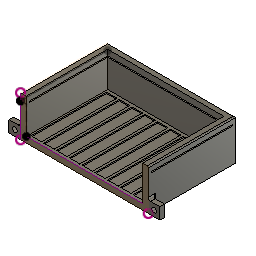
LIght box v2 (Autodesk Fusion 360 design; units mm, degrees)
Autodesk Fusion 360 part; units mm, degrees
sketch "Box base" plane through (0, 0, 0) normal (0, 1, 0) x (1, 0, 0)
  line L0 (55, -40) -> (-55, -40)
  line L1 (-55, -40) -> (-55, 40)
  line L2 (-55, 40) -> (55, 40)
  line L3 (55, 40) -> (55, -40)
  line L4 (55, -40) -> (-55, 40) construction
  line L5 (-55, -40) -> (55, 40) construction
  dimension "d3" = 110
  dimension "d4" = 80
extrude "Extrude2" add sketch "Box base" along normal blind 35
sketch "Center box" plane through (0, 35, 0) normal (0, 1, 0) x (-1, 0, 0)
  line L0 (-55, -40) -> (55, -40)
  line L1 (55, -40) -> (55, 40)
  line L2 (55, 40) -> (-55, 40)
  line L3 (-55, 40) -> (-55, -40)
  line L4 (-50, 35) -> (50, 35)
  line L5 (50, 35) -> (50, -35)
  line L6 (50, -35) -> (-50, -35)
  line L7 (-50, -35) -> (-50, 35)
  line L8 (-50, 35) -> (50, -35) construction
  line L9 (50, 35) -> (-50, -35) construction
  dimension "d9" = 100
  dimension "d10" = 70
extrude "Extrude3" cut sketch "Center box" against normal blind 30 contours L4 L5 L6 L7
sketch "open one end" plane through (0, 0, 40) normal (0, 0, 1) x (1, 0, 0)
  line L0 (-55, 0) -> (55, 0)
  line L1 (55, 0) -> (55, 35)
  line L2 (55, 35) -> (-55, 35)
  line L3 (-55, 35) -> (-55, 0)
  line L4 (-55, 35) -> (55, 35)
  line L5 (55, 35) -> (55, 0)
  line L6 (55, 0) -> (-55, 0)
  line L7 (-55, 0) -> (-55, 35)
extrude "Extrude4" cut sketch "open one end" against normal blind 5
sketch "line marker for slit" plane through (0, 0, 35) normal (0, 0, 1) x (1, 0, 0)
  line L0 (-50, 5) -> (-50, 35)
  line L1 (-50, 35) -> (-55, 35)
  line L2 (-55, 35) -> (-55, 0)
  line L3 (-55, 0) -> (55, 0)
  line L4 (55, 0) -> (55, 35)
  line L5 (55, 35) -> (50, 35)
  line L6 (50, 35) -> (50, 5)
  line L7 (-50, 5) -> (-50, 29) construction
  line L8 (-50, 29) -> (-55, 29) construction
  line L9 (-55, 0) -> (-55, 35)
  line L10 (50, 5) -> (-50, 5)
  dimension "d21" = 24
  measures "d21" distance of origin
sketch "Slit for diffuser" plane through (-55, 0, 0) normal (-1, 0, 0) x (0, 0, 1)
  line L0 (35, 0) -> (35, 35)
  line L1 (35, 35) -> (-40, 35)
  line L2 (-40, 35) -> (-40, 0)
  line L3 (-40, 0) -> (35, 0)
  line L4 (-40, 29) -> (35, 29) construction
  line L5 (-37.5, 30) -> (32.5, 30)
  line L6 (32.5, 30) -> (32.5, 29)
  line L7 (32.5, 29) -> (-37.5, 29)
  line L8 (-37.5, 29) -> (-37.5, 30)
  dimension "d22" = 70
  dimension "d23" = 1
extrude "Extrude6" cut sketch "Slit for diffuser" against normal up to surface (110 mm away) contours L5 L6 L7 L8
sketch "IR strip pads" plane through (0, 35, 0) normal (0, 1, 0) x (-1, 0, 0)
  line L0 (4.5, -32.5) -> (-4.5, -32.5)
  line L1 (-4.5, -32.5) -> (-4.5, 32.5)
  line L2 (-4.5, 32.5) -> (4.5, 32.5)
  line L3 (4.5, 32.5) -> (4.5, -32.5)
  line L4 (4.5, -32.5) -> (-4.5, 32.5) construction
  line L5 (-4.5, -32.5) -> (4.5, 32.5) construction
  dimension "d28" = 9
  dimension "d29" = 65
extrude "Extrude7" cut sketch "IR strip pads" against normal blind 31
pattern_linear "R-Pattern1" count 9 spacing 11 along (-1, 0, 0) both ways of "Extrude7"
sketch "nut holder" plane through (0, 0, 35) normal (0, 0, 1) x (1, 0, 0)
  line L0 (55, 10) -> (65, 10)
  line L1 (65, 10) -> (65, 0)
  line L2 (65, 0) -> (55, 0)
  line L3 (55, 0) -> (55, 10)
  circle A0 centre (60, 5) radius 2
  line L4 (60, 10) -> (60, 0) construction
  line L5 (65, 5) -> (55, 5) construction
  dimension "d36" = 10
  dimension "d37" = 10
  dimension "d43" = 4
  measures "d37" distance of origin
  measures "d43" diameter of A0
extrude "Extrude8" add sketch "nut holder" against normal blind 4 contours L0 L1 L2 L3 | A0
extrude "Extrude9" cut sketch "nut holder" against normal blind 4 contours A0
fillet "Fillet1" radius 2 2 edges at (55, 10, 33) (55, 5, 31)
mirror "Mirror2" about plane through (0, 0, 0) normal (1, 0, 0) of "Extrude8", "Extrude9"
fillet "Fillet3" radius 2 2 edges at (-55, 10, 33) (-55, 5, 31)
fillet "Fillet4" radius 1 3 edges at (0, 35, -40) (-55, 35, -2.5) (55, 35, -2.5)
